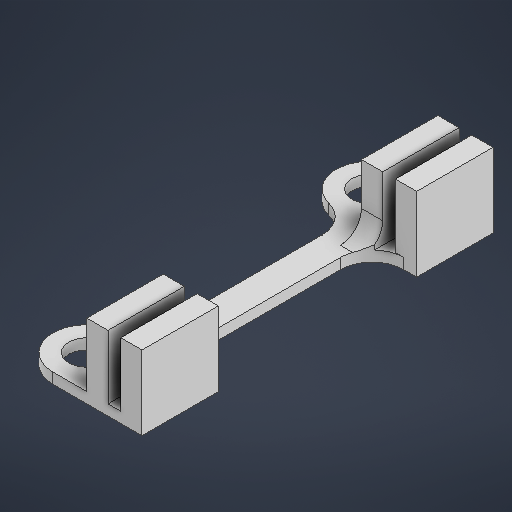
# Autodesk Inventor part: esp holder
Saved by Autodesk Inventor 2026 (Build 300175000, 175)
## iProperties
Created: 2025-06-20
Part Number: esp holder
Material: Všeobecné
Document SubType Name: Modeling
Designer: vadim
Density: 1 g/cm^3
Appearance: Výchozí
Author: vadim
Autodesk Inventor part; units mm, degrees
ref_plane "YZ Plane" through (0, 0, 0) normal (1, 0, 0) x (0, 1, 0)
ref_plane "XZ Plane" through (0, 0, 0) normal (0, 1, 0) x (-1, 0, 0)
ref_plane "XY Plane" through (0, 0, 0) normal (0, 0, 1) x (1, 0, 0)
sketch "Náčrt1" plane through (0, 0, 0) normal (0, 1, 0) x (-1, 0, 0)
  line L0 (0, 0) -> (10.4898, 0)
  line L1 (6.7377, 13.35) -> (6.7377, -13.35)
  line L2 (4.2782, 13.5) -> (4.2782, -13.5)
  line L3 (3.5377, 9.35) -> (3.5377, -9.35)
  circle A0 centre (6.7377, -13.35) radius 1.7
  line L4 (3.5377, -9.35) -> (1.5377, -9.35)
  line L5 (1.5377, -9.35) -> (1.5377, -16.55)
  line L6 (1.5377, -16.55) -> (3.5377, -16.55)
  line L7 (3.5377, -16.55) -> (3.5377, -9.35)
  arc A1 (6.7377, -16.55) -> (6.7377, -10.15) centre (6.7377, -13.35) ccw
  line L8 (6.7377, -10.15) -> (3.5377, -10.15)
  line L9 (6.7377, -16.55) -> (1.5377, -16.55)
  line L10 (0.3377, -9.35) -> (-1.6623, -9.35)
  line L11 (-1.6623, -9.35) -> (-1.6623, -16.55)
  line L12 (-1.6623, -16.55) -> (0.3377, -16.55)
  line L13 (0.3377, -16.55) -> (0.3377, -9.35)
  line L14 (-1.6623, -16.55) -> (-1.6623, -16.55)
  line L15 (-1.6623, -16.55) -> (1.5377, -16.55)
  line L16 (1.5377, -9.35) -> (0.3377, -9.35)
  line L17 (2.5377, -10.15) -> (5.2449, -10.15)
  line L18 (5.2449, -10.15) -> (5.2449, 0)
  line L19 (5.2449, 0) -> (2.5377, 0)
  line L20 (2.5377, 0) -> (2.5377, -10.15)
  point P0 (2.5377, -9.35)
  dimension "d0" = 26.7
  dimension "d1" = 27
  dimension "d2" = 18.7
  dimension "d4" = 3.4
  dimension "d5" = 2
  dimension "d7" = 1.5
  dimension "d9" = 2
  dimension "d11" = 1.2
  constraints: 42 end point, 7 parallel, 4 collinear, 4 horizontal, 4 perpendicular, 4 point on line, 4 vertical, 3 symmetric about line, 3 tangent, 2 centre point, 2 point on circle, 1 coincident, 1 midpoint
  measures "d0" distance of L1.start L1.end
  measures "d1" distance of L2.start L2.end
  measures "d2" distance of L3.start L3.end
  measures "d4" diameter of A0
  measures "d5" distance of L6.end L5.end
  measures "d7" radial gap between concentric circles of A0 A1
  measures "d9" distance of L12.end L11.end
  measures "d11" distance between parallel lines of L13 L5
extrude "Vysunutí1" add sketch "Náčrt1" along normal blind 1 contours L0 L3 L4 L20 | L0 L2 L8 L7 L3 | L4 L7 L17 L20 | L0 L18 L8 L2 | L5 L15 L13 L16 | L8 A1 L9 L7
extrude "Vysunutí2" add sketch "Náčrt1" along normal blind 7 contours L20 L17 L7 L6 L5 L4 | L4 L7 L17 L20 | L13 L12 L11 L10
mirror "Zrcadlit1" about plane through (-5.2449, 0, 0) normal (0, 0, 1) of "Vysunutí2", "Vysunutí1"
fillet "Zaoblení1" radius 3 2 edges at (-2.5377, 0.5, 9.35) (-2.5377, 0.5, -9.35)
fillet "Zaoblení2" radius 3 2 edges at (-5.2449, 0.5, 10.15) (-5.2449, 0.5, -10.15)
fillet "Zaoblení3" radius 2 2 edges at (-2.5377, 1, 9.35) (-2.5377, 1, -9.35)
